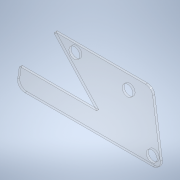
# Autodesk Inventor part: 2021 Intake Panels
Saved by Autodesk Inventor 2021.1 (Build 251245000, 245)
## iProperties
Created: 2021-01-29
Part Number: 2021 Intake Panels
Material: Polycarbonate, Clear
Document SubType Name: Modeling
Designer: aidan
Density: 1.2 g/cm^3
Appearance: Polycarbonate - Clear
Author: aidan
Autodesk Inventor part; units mm, degrees
ref_plane "YZ Plane" through (0, 0, 0) normal (1, 0, 0) x (0, 1, 0)
ref_plane "XZ Plane" through (0, 0, 0) normal (0, 1, 0) x (-1, 0, 0)
ref_plane "XY Plane" through (0, 0, 0) normal (0, 0, 1) x (1, 0, 0)
sketch "Sketch1" plane through (0, 0, 0) normal (0, 0, 1) x (1, 0, 0)
  line L0 (-177.5744, 25.4) -> (-152.1744, 203.2)
  line L1 (-152.1744, 203.2) -> (178.0256, 203.2)
  line L2 (178.0256, 203.2) -> (203.4256, 25.4)
  line L3 (203.4256, 25.4) -> (-177.5744, 25.4)
  circle A0 centre (114.3, 165.1) radius 14.2875
  circle A1 centre (-25.4, 180.975) radius 14.2875
  circle A2 centre (177.8, 47.625) radius 14.2875
  circle A3 centre (505.2413, 166.6875) radius 88.9 construction
  line L4 (-713.704, 0) -> (0, 0) construction
  line L5 (0, 0) -> (0, -152.4) construction
  line L6 (0, -152.4) -> (-713.704, -152.4) construction
  line L7 (-713.704, -152.4) -> (-713.704, 0) construction
  circle A4 centre (177.8, 47.625) radius 50.8 construction
  line L8 (0, -152.4) -> (745.4464, -152.4) construction
  dimension "d0" = 28.575
  dimension "d1" = 22.225
  dimension "d2" = 22.225
  dimension "d7" = 177.8
  dimension "d8" = 152.4
  dimension "d9" = 101.6
  dimension "d11" = 177.8
  dimension "d12" = 25.4
  dimension "d13" = 177.8
  dimension "d14" = 22.225
  dimension "d15" = 203.2
  dimension "d16" = 38.1
  dimension "d17" = 63.5
  dimension "d18" = 381
  dimension "d19" = 330.2
  constraints: 18 end point, 5 centre point, 4 horizontal, 2 coincident, 2 equal radius, 2 parallel, 1 equal length, 1 perpendicular
  measures "d0" diameter of A1
  measures "d1" distance from line of A2.centre L3
  measures "d2" distance from line of L2 A2.centre
  measures "d7" diameter of A3
  measures "d8" distance of L4.end L5.end
  measures "d9" diameter of A4
  measures "d11" horizontal distance of A2.centre point (0, 0)
  measures "d12" distance between parallel lines of L3 L4
  measures "d13" distance between parallel lines of L3 L1
  measures "d14" distance from line of L1 A1.centre
  measures "d15" horizontal distance of A2.centre A1.centre
  measures "d16" distance from line of L1 A0.centre
  measures "d17" horizontal distance of A4.centre A0.centre
  measures "d18" distance of L2.end L0.start
  measures "d19" distance of L0.end L1.end
extrude "Extrusion1" add sketch "Sketch1" along normal blind 5.588
fillet "Fillet1" radius 19.05 4 edges at (203.4256, 25.4, 2.794) (178.0256, 203.2, 2.794) (-152.1744, 203.2, 2.794) (-177.5744, 25.4, 2.794)
sketch "Sketch2" plane through (0, 0, 5.588) normal (0, 0, 1) x (1, 0, 0)
  line L0 (-154.5109, 186.8441) -> (-174.4681, 47.1441) projected
  line L1 (-170.014, 78.3223) -> (33.186, 78.3223)
  line L2 (33.186, 78.3223) -> (-82.5653, 203.2)
  line L3 (161.5037, 203.2) -> (-135.6524, 203.2) projected
  line L4 (-82.5653, 203.2) -> (-152.1744, 203.2)
  line L5 (-152.1744, 203.2) -> (-170.014, 78.3223)
  point P0 (0, 0)
  dimension "d23" = 203.2
  constraints: 8 end point, 3 point on line, 1 collinear, 1 horizontal
  measures "d23" distance of L1.start L1.end
extrude "Extrusion2" cut sketch "Sketch2" against normal through all
fillet "Fillet2" radius 3.175 2 edges at (-170.014, 78.3223, 2.794) (-82.5653, 203.2, 2.794)
body "Solid1"
